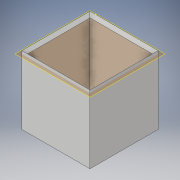
# Autodesk Inventor part: insulationbox
Saved by Autodesk Inventor 2018 (Build 220112000, 112)
## iProperties
Created: 2019-02-19
Part Number: insulationbox
Material: Generic
Document SubType Name: Modeling
Designer: F8PLTW
Density: 1 g/cm^3
Appearance: Default
Author: F8PLTW
Autodesk Inventor part; units mm, degrees
ref_plane "YZ Plane" through (0, 0, 0) normal (1, 0, 0) x (0, 1, 0)
ref_plane "XZ Plane" through (0, 0, 0) normal (0, 1, 0) x (-1, 0, 0)
ref_plane "XY Plane" through (0, 0, 0) normal (0, 0, 1) x (1, 0, 0)
sketch "Sketch1" plane through (0, 0, 0) normal (0, 0, 1) x (1, 0, 0)
  line L0 (-12.9018, 8.1017) -> (137.0982, 8.1017)
  line L1 (137.0982, 8.1017) -> (137.0982, -141.8983)
  line L2 (137.0982, -141.8983) -> (-12.9018, -141.8983)
  line L3 (-12.9018, -141.8983) -> (-12.9018, 8.1017)
  point P0 (0, 0)
  dimension "d0" = 150
  dimension "d1" = 150
  constraints: 8 end point, 2 parallel, 1 horizontal, 1 perpendicular
  measures "d0" distance of L1.end L2.end
  measures "d1" distance of L0.end L1.end
extrude "Extrusion1" add sketch "Sketch1" along normal blind 150
sketch "Sketch2" plane through (-12.9018, 8.1017, 0) normal (0, 1, 0) x (1, 0, 0)
  point P0 (12.9018, 0)
ref_plane "Work Plane1" through (-12.9018, 1.7517, 0) normal (0, 1, 0) x (1, 0, 0)
sketch "Sketch3" plane through (-12.9018, 1.7517, 0) normal (0, 1, 0) x (1, 0, 0)
  line L0 (6.35, -143.65) -> (143.65, -143.65)
  line L1 (143.65, -143.65) -> (143.65, -6.35)
  line L2 (143.65, -6.35) -> (6.35, -6.35)
  line L3 (6.35, -6.35) -> (6.35, -143.65)
  line L4 (150, -150) -> (0, -150) projected
  line L5 (0, 0) -> (0, -150) projected
  point P0 (12.9018, 0)
  dimension "d5" = 137.3
  dimension "d6" = 137.3
  dimension "d7" = 6.35
  dimension "d8" = 6.35
  constraints: 8 end point, 2 parallel, 1 horizontal, 1 perpendicular
  measures "d5" distance of L2.end L1.end
  measures "d6" distance of L1.end L0.end
  measures "d7" distance between parallel lines of L4 L0
  measures "d8" distance between parallel lines of L5 L3
loft "Loft1" cut profiles "Sketch3" section 1 edges at (62.0982, 8.1017, 0) (-12.9018, 8.1017, 75) (62.0982, 8.1017, 150) (137.0982, 8.1017, 75)
sketch "Sketch4" plane through (-6.5518, 1.7517, 6.35) normal (0, 1, 0) x (1, 0, 0)
  line L0 (0, -137.3) -> (137.3, -137.3) projected
  line L1 (137.3, -137.3) -> (137.3, 0) projected
  line L2 (0, -137.3) -> (137.3, -137.3)
  line L3 (137.3, -137.3) -> (137.3, 0)
  line L4 (137.3, 0) -> (0, 0)
  line L5 (0, 0) -> (0, -137.3)
  point P0 (6.5518, 6.35)
  constraints: 8 end point, 2 parallel, 1 horizontal, 1 perpendicular
extrude "Extrusion2" cut sketch "Sketch4" against normal blind 137.3
body "Solid1"
